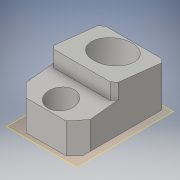
# Autodesk Inventor part: led_holder_v13
Saved by Autodesk Inventor 2016 (Build 200138000, 138)
## iProperties
Created: 2018-09-25
Part Number: led_holder_v13
Material: Generic
Document SubType Name: Modeling
Designer: tar
Density: 1 g/cm^3
Appearance: Default
Author: tar
Autodesk Inventor part; units mm, degrees
ref_plane "YZ Plane" through (0, 0, 0) normal (1, 0, 0) x (0, 1, 0)
ref_plane "XZ Plane" through (0, 0, 0) normal (0, 1, 0) x (-1, 0, 0)
ref_plane "XY Plane" through (0, 0, 0) normal (0, 0, 1) x (1, 0, 0)
sketch "Skizze5" plane through (0, 0, 0) normal (1, 0, 0) x (0, 1, 0)
  line L0 (0, 0) -> (0, 0)
  line L1 (0, 0) -> (4.4737, 0.486)
  line L2 (4.4737, 0.486) -> (10.9319, -0.2498)
  line L3 (10.9319, -0.2498) -> (10.9319, -0.2498)
  line L4 (10.9319, -0.2498) -> (10.9319, 5.2858)
  line L5 (10.9319, 5.2858) -> (4.4737, 6.0216)
  line L6 (0, 3.5206) -> (0, 0)
  line L7 (0, 3.5206) -> (4.4737, 4.0066)
  line L8 (4.4737, 8.0188) -> (4.4737, 2.9641) construction
  line L9 (4.4737, 6.0216) -> (4.4737, 4.0066)
  dimension "d21" = 0
  dimension "d22" = 6.2
  dimension "d23" = 6.5
  dimension "d24" = 4.5
  dimension "d25" = 6.5
  dimension "d26" = 5.5
  dimension "d27" = 3.5
  constraints: 20 end point, 4 parallel, 4 point on line, 2 perpendicular, 1 horizontal, 1 midpoint, 1 vertical
  measures "d21" distance of L0.start L0.end
  measures "d22" angle of L1 L0
  measures "d23" angle of L2 L3
  measures "d24" distance of L0.end L1.end
  measures "d25" distance of L1.end L2.end
  measures "d26" distance between parallel lines of L5 L2
  measures "d27" distance between parallel lines of L1 L7
extrude "Extrusion3" add sketch "Skizze5" along normal blind 8
sketch "Skizze6" plane through (8, 10.9319, -0.2498) normal (0, -0.1132, -0.9936) x (-1, 0, 0)
  circle A0 centre (4, -3.25) radius 2.425
  line L0 (4, 0.2781) -> (4, -10.3498)
  line L1 (-1.6335, -3.25) -> (9.1615, -3.25)
  line L2 (8, -6.5) -> (8, 0) projected
  line L3 (8, 0) -> (0, 0) projected
  point P0 (8, -10.8899)
  point P1 (8, -1.2477)
  point P2 (4, -0.9743)
  point P3 (8, -3.25)
  point P4 (4, 0)
  dimension "d30" = 4.85
  constraints: 5 point on line, 4 end point, 2 midpoint, 1 centre point, 1 horizontal, 1 vertical
  measures "d30" diameter of A0
extrude "Extrusion4" cut sketch "Skizze6" against normal through all contours L1 L0 A0 | A0 L0 L1 | L0 L1 A0 | A0 L1 L0
sketch "Skizze7" plane through (8, 4.4737, 0.486) normal (0, 0.108, -0.9942) x (-1, 0, 0)
  line L0 (-0.5646, -2.25) -> (9.8389, -2.25)
  line L1 (4, -0.832) -> (4, -8.1647)
  circle A0 centre (4, -2.25) radius 1.65
  line L2 (8, -4.5) -> (8, 0) projected
  line L3 (8, -4.5) -> (0, -4.5) projected
  point P0 (4, -5.6763)
  point P1 (8, -2.25)
  point P2 (8, -2.25)
  point P3 (4, -4.5)
  dimension "d33" = 3.3
  constraints: 6 point on line, 4 end point, 2 midpoint, 1 centre point, 1 horizontal, 1 vertical
  measures "d33" diameter of A0
extrude "Extrusion5" cut sketch "Skizze7" against normal through all contours A0 L0 | L0 L1 A0 | L0 A0 L1
chamfer "Fase2" distance 0.5 angle 45 4 edges at (8, 10.9319, 2.518) (0, 10.9319, 2.518) (8, 4.4737, 5.0141) (0, 4.4737, 5.0141)
ref_plane "Arbeitsebene3" through (0, 10.9319, -0.2498) normal (0, 0, 1) x (1, 0, 0)
sketch "Skizze11" plane through (0, 10.9319, -0.2498) normal (0, 0, 1) x (1, 0, 0)
  line L0 (0.5, 0) -> (7.5, 0) projected
  line L1 (8, -0.5) -> (7.5, 0) projected
  line L2 (8, -6.4582) -> (8, -0.5) projected
  line L3 (8, -10.9319) -> (8, -6.4582) projected
  line L4 (0, -10.9319) -> (8, -10.9319) projected
  line L5 (0, -10.9319) -> (0, -6.4582) projected
  line L6 (0, -6.4582) -> (0, -0.5) projected
  line L7 (0.5, 0) -> (0, -0.5) projected
extrude "Extrusion9" add sketch "Skizze11" along normal blind 1
sketch "Skizze12" plane through (0.5, 4.4737, 6.0216) normal (0, 0.1132, 0.9936) x (1, 0, 0)
  circle A0 centre (3.5, 3.8766) radius 2.425 projected
  point P0 (-0.5, -3.7633)
extrude "Extrusion10" cut sketch "Skizze12" against normal through all
sketch "Skizze13" plane through (0, 0, 3.5206) normal (0, -0.108, 0.9942) x (1, 0, 0)
  circle A0 centre (4, 1.8698) radius 1.65 projected
  point P0 (0, -0.3802)
extrude "Extrusion11" cut sketch "Skizze13" against normal through all
chamfer "Fase4" distance 0.5 angle 45 3 edges at (8, 5.2159, -0.2498) (4, 10.9319, -0.2498) (0, 5.2159, -0.2498)
chamfer "Fase5" distance 1.5 angle 45 2 edges at (8, 0, 1.8854) (0, 0, 1.8854)
